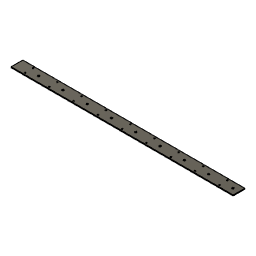
16 mm Rail Plate v3 (Autodesk Fusion 360 design; units mm, degrees)
Autodesk Fusion 360 part; units mm, degrees
sketch "Sketch1" plane through (0, 0, 0) normal (0, 0, 1) x (1, 0, 0)
  line L0 (0, 0) -> (914.4, 0)
  line L1 (914.4, 0) -> (914.4, 48)
  line L2 (914.4, 48) -> (0, 48)
  line L3 (0, 48) -> (0, 0)
  dimension "d1" = 48
  dimension "d2" = 914.4
  constraint horizontal L0
  constraint vertical L1
  constraint horizontal L2
  constraint vertical L3
  constraint coincident L0.start L3.end
  measures "d1" distance of L0.start L2.end
  measures "d2" distance of L1.end L2.end
extrude "Extrude1" add sketch "Sketch1" along normal blind 3.175
sketch "Sketch2" plane through (0, 0, 3.175) normal (0, 0, 1) x (-1, 0, 0)
  line L0 (0, -48) -> (0, 0)
  line L1 (0, 0) -> (-914.4, 0)
  line L2 (-914.4, 0) -> (-914.4, -48)
  line L3 (-914.4, -48) -> (0, -48)
  line L4 (0, -48) -> (-50, -48)
  line L5 (-50, -48) -> (-50, -40.5)
  circle A0 centre (-50, -40.5) radius 2.75
  line L6 (-914.4, -48) -> (-914.4, -24)
  line L7 (-914.4, -24) -> (-889.4, -24)
  circle A1 centre (-889.4, -24) radius 4
  circle A2 centre (-789.4, -24) radius 4
  circle A3 centre (-689.4, -24) radius 4
  circle A4 centre (-589.4, -24) radius 4
  circle A5 centre (-489.4, -24) radius 4
  circle A6 centre (-389.4, -24) radius 4
  circle A7 centre (-289.4, -24) radius 4
  circle A8 centre (-189.4, -24) radius 4
  circle A9 centre (-89.4, -24) radius 4
  circle A10 centre (-150, -40.5) radius 2.75
  circle A11 centre (-250, -40.5) radius 2.75
  circle A12 centre (-350, -40.5) radius 2.75
  circle A13 centre (-450, -40.5) radius 2.75
  circle A14 centre (-550, -40.5) radius 2.75
  circle A15 centre (-650, -40.5) radius 2.75
  circle A16 centre (-750, -40.5) radius 2.75
  circle A17 centre (-850, -40.5) radius 2.75
  circle A18 centre (-50, -7.5) radius 2.75
  circle A19 centre (-150, -7.5) radius 2.75
  circle A20 centre (-250, -7.5) radius 2.75
  circle A21 centre (-350, -7.5) radius 2.75
  circle A22 centre (-450, -7.5) radius 2.75
  circle A23 centre (-550, -7.5) radius 2.75
  circle A24 centre (-650, -7.5) radius 2.75
  circle A25 centre (-750, -7.5) radius 2.75
  circle A26 centre (-850, -7.5) radius 2.75
  dimension "d5" = 50
  dimension "d6" = 7.5
  dimension "d7" = 5.5
  dimension "d10" = -100
  dimension "d11" = 33
  dimension "d12" = 25
  dimension "d13" = 8
  dimension "d16" = 100
  dimension "d17" = 0
  constraint coincident L0.start L3.end
  constraint perpendicular L0 L4
  constraint perpendicular L4 L5
  constraint coincident L5.end A0.centre
  constraint coincident L2.end L3.start
  constraint midpoint L2 L6.end
  constraint perpendicular L2 L7
  constraint coincident L7.end A1.centre
  measures "d5" distance of L0.start L4.end
  measures "d6" distance of L4.end L5.end
  measures "d7" diameter of A0
  measures "d12" distance of L6.end L7.end
  measures "d13" diameter of A1
extrude "Extrude2" cut sketch "Sketch2" against normal blind 60.31 contours A0 | A1 | A2 | A3 | A4 | A5 | A6 | A7 | A8 | A9 | A10 | A11 | A12 | A13 | A14 | A15 | A16 | A17 | A18 | A19 | A20 | A21 | A22 | A23 | A24 | A25 | A26
